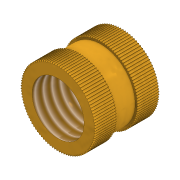
# Autodesk Inventor part: M5 7mm OD 8mm Deep Threaded Insert
Saved by Autodesk Inventor 2020 (Build 240168000, 168)
## iProperties
Created: 2021-07-20
Part Number: M5 7mm OD 8mm Deep Threaded Insert
Material: Generic
Document SubType Name: Modeling
Designer: Coy
Density: 1 g/cm^3
Appearance: Weld - Brass
Author: Coy
Autodesk Inventor part; units mm, degrees
ref_plane "YZ Plane" through (0, 0, 0) normal (1, 0, 0) x (0, 1, 0)
ref_plane "XZ Plane" through (0, 0, 0) normal (0, 1, 0) x (-1, 0, 0)
ref_plane "XY Plane" through (0, 0, 0) normal (0, 0, 1) x (1, 0, 0)
sketch "Sketch1" plane through (0, 0, 0) normal (0, 0, 1) x (1, 0, 0)
  circle A0 centre (0, 0) radius 2.45
  circle A1 centre (0, 0) radius 3.5
  arc A2 (-0.1, 3.4986) -> (0.1, 3.4986) centre (0, 3.5) ccw
  arc A3 (-0.3195, 3.4854) -> (-0.1199, 3.4979) centre (-0.2198, 3.4931) ccw
  arc A4 (-0.5377, 3.4585) -> (-0.3393, 3.4835) centre (-0.4387, 3.4724) ccw
  arc A5 (-0.7538, 3.4179) -> (-0.5573, 3.4553) centre (-0.6558, 3.438) ccw
  arc A6 (-0.9669, 3.3638) -> (-0.7732, 3.4135) centre (-0.8704, 3.39) ccw
  arc A7 (-1.1762, 3.2964) -> (-0.986, 3.3582) centre (-1.0816, 3.3287) ccw
  arc A8 (-1.3809, 3.2161) -> (-1.1949, 3.2897) centre (-1.2884, 3.2542) ccw
  arc A9 (-1.5801, 3.123) -> (-1.3991, 3.2082) centre (-1.4902, 3.1669) ccw
  arc A10 (-1.7731, 3.0177) -> (-1.5978, 3.114) centre (-1.6861, 3.0671) ccw
  arc A11 (-1.9591, 2.9004) -> (-1.7902, 3.0075) centre (-1.8754, 2.9551) ccw
  arc A12 (-2.1373, 2.7716) -> (-1.9755, 2.8892) centre (-2.0572, 2.8316) ccw
  arc A13 (-2.3071, 2.632) -> (-2.153, 2.7594) centre (-2.231, 2.6968) ccw
  arc A14 (-2.4678, 2.4819) -> (-2.322, 2.6188) centre (-2.3959, 2.5514) ccw
  arc A15 (-2.6188, 2.322) -> (-2.4819, 2.4678) centre (-2.5514, 2.3959) ccw
  arc A16 (-2.7594, 2.153) -> (-2.632, 2.3071) centre (-2.6968, 2.231) ccw
  arc A17 (-2.8892, 1.9755) -> (-2.7716, 2.1373) centre (-2.8316, 2.0572) ccw
  arc A18 (-3.0075, 1.7902) -> (-2.9004, 1.9591) centre (-2.9551, 1.8754) ccw
  arc A19 (-3.114, 1.5978) -> (-3.0177, 1.7731) centre (-3.0671, 1.6861) ccw
  arc A20 (-3.2082, 1.3991) -> (-3.123, 1.5801) centre (-3.1669, 1.4902) ccw
  arc A21 (-3.2897, 1.1949) -> (-3.2161, 1.3809) centre (-3.2542, 1.2884) ccw
  arc A22 (-3.3582, 0.986) -> (-3.2964, 1.1762) centre (-3.3287, 1.0816) ccw
  arc A23 (-3.4135, 0.7732) -> (-3.3638, 0.9669) centre (-3.39, 0.8704) ccw
  arc A24 (-3.4553, 0.5573) -> (-3.4179, 0.7538) centre (-3.438, 0.6558) ccw
  arc A25 (-3.4835, 0.3393) -> (-3.4585, 0.5377) centre (-3.4724, 0.4387) ccw
  arc A26 (-3.4979, 0.1199) -> (-3.4854, 0.3195) centre (-3.4931, 0.2198) ccw
  arc A27 (-3.4986, -0.1) -> (-3.4986, 0.1) centre (-3.5, 0) ccw
  arc A28 (-3.4854, -0.3195) -> (-3.4979, -0.1199) centre (-3.4931, -0.2198) ccw
  arc A29 (-3.4585, -0.5377) -> (-3.4835, -0.3393) centre (-3.4724, -0.4387) ccw
  arc A30 (-3.4179, -0.7538) -> (-3.4553, -0.5573) centre (-3.438, -0.6558) ccw
  arc A31 (-3.3638, -0.9669) -> (-3.4135, -0.7732) centre (-3.39, -0.8704) ccw
  arc A32 (-3.2964, -1.1762) -> (-3.3582, -0.986) centre (-3.3287, -1.0816) ccw
  arc A33 (-3.2161, -1.3809) -> (-3.2897, -1.1949) centre (-3.2542, -1.2884) ccw
  arc A34 (-3.123, -1.5801) -> (-3.2082, -1.3991) centre (-3.1669, -1.4902) ccw
  arc A35 (-3.0177, -1.7731) -> (-3.114, -1.5978) centre (-3.0671, -1.6861) ccw
  arc A36 (-2.9004, -1.9591) -> (-3.0075, -1.7902) centre (-2.9551, -1.8754) ccw
  arc A37 (-2.7716, -2.1373) -> (-2.8892, -1.9755) centre (-2.8316, -2.0572) ccw
  arc A38 (-2.632, -2.3071) -> (-2.7594, -2.153) centre (-2.6968, -2.231) ccw
  arc A39 (-2.4819, -2.4678) -> (-2.6188, -2.322) centre (-2.5514, -2.3959) ccw
  arc A40 (-2.322, -2.6188) -> (-2.4678, -2.4819) centre (-2.3959, -2.5514) ccw
  arc A41 (-2.153, -2.7594) -> (-2.3071, -2.632) centre (-2.231, -2.6968) ccw
  arc A42 (-1.9755, -2.8892) -> (-2.1373, -2.7716) centre (-2.0572, -2.8316) ccw
  arc A43 (-1.7902, -3.0075) -> (-1.9591, -2.9004) centre (-1.8754, -2.9551) ccw
  arc A44 (-1.5978, -3.114) -> (-1.7731, -3.0177) centre (-1.6861, -3.0671) ccw
  arc A45 (-1.3991, -3.2082) -> (-1.5801, -3.123) centre (-1.4902, -3.1669) ccw
  arc A46 (-1.1949, -3.2897) -> (-1.3809, -3.2161) centre (-1.2884, -3.2542) ccw
  arc A47 (-0.986, -3.3582) -> (-1.1762, -3.2964) centre (-1.0816, -3.3287) ccw
  arc A48 (-0.7732, -3.4135) -> (-0.9669, -3.3638) centre (-0.8704, -3.39) ccw
  arc A49 (-0.5573, -3.4553) -> (-0.7538, -3.4179) centre (-0.6558, -3.438) ccw
  arc A50 (-0.3393, -3.4835) -> (-0.5377, -3.4585) centre (-0.4387, -3.4724) ccw
  arc A51 (-0.1199, -3.4979) -> (-0.3195, -3.4854) centre (-0.2198, -3.4931) ccw
  arc A52 (0.1, -3.4986) -> (-0.1, -3.4986) centre (0, -3.5) ccw
  arc A53 (0.3195, -3.4854) -> (0.1199, -3.4979) centre (0.2198, -3.4931) ccw
  arc A54 (0.5377, -3.4585) -> (0.3393, -3.4835) centre (0.4387, -3.4724) ccw
  arc A55 (0.7538, -3.4179) -> (0.5573, -3.4553) centre (0.6558, -3.438) ccw
  arc A56 (0.9669, -3.3638) -> (0.7732, -3.4135) centre (0.8704, -3.39) ccw
  arc A57 (1.1762, -3.2964) -> (0.986, -3.3582) centre (1.0816, -3.3287) ccw
  arc A58 (1.3809, -3.2161) -> (1.1949, -3.2897) centre (1.2884, -3.2542) ccw
  arc A59 (1.5801, -3.123) -> (1.3991, -3.2082) centre (1.4902, -3.1669) ccw
  arc A60 (1.7731, -3.0177) -> (1.5978, -3.114) centre (1.6861, -3.0671) ccw
  arc A61 (1.9591, -2.9004) -> (1.7902, -3.0075) centre (1.8754, -2.9551) ccw
  arc A62 (2.1373, -2.7716) -> (1.9755, -2.8892) centre (2.0572, -2.8316) ccw
  arc A63 (2.3071, -2.632) -> (2.153, -2.7594) centre (2.231, -2.6968) ccw
  arc A64 (2.4678, -2.4819) -> (2.322, -2.6188) centre (2.3959, -2.5514) ccw
  arc A65 (2.6188, -2.322) -> (2.4819, -2.4678) centre (2.5514, -2.3959) ccw
  arc A66 (2.7594, -2.153) -> (2.632, -2.3071) centre (2.6968, -2.231) ccw
  arc A67 (2.8892, -1.9755) -> (2.7716, -2.1373) centre (2.8316, -2.0572) ccw
  arc A68 (3.0075, -1.7902) -> (2.9004, -1.9591) centre (2.9551, -1.8754) ccw
  arc A69 (3.114, -1.5978) -> (3.0177, -1.7731) centre (3.0671, -1.6861) ccw
  arc A70 (3.2082, -1.3991) -> (3.123, -1.5801) centre (3.1669, -1.4902) ccw
  arc A71 (3.2897, -1.1949) -> (3.2161, -1.3809) centre (3.2542, -1.2884) ccw
  arc A72 (3.3582, -0.986) -> (3.2964, -1.1762) centre (3.3287, -1.0816) ccw
  arc A73 (3.4135, -0.7732) -> (3.3638, -0.9669) centre (3.39, -0.8704) ccw
  arc A74 (3.4553, -0.5573) -> (3.4179, -0.7538) centre (3.438, -0.6558) ccw
  arc A75 (3.4835, -0.3393) -> (3.4585, -0.5377) centre (3.4724, -0.4387) ccw
  arc A76 (3.4979, -0.1199) -> (3.4854, -0.3195) centre (3.4931, -0.2198) ccw
  arc A77 (3.4986, 0.1) -> (3.4986, -0.1) centre (3.5, 0) ccw
  arc A78 (3.4854, 0.3195) -> (3.4979, 0.1199) centre (3.4931, 0.2198) ccw
  arc A79 (3.4585, 0.5377) -> (3.4835, 0.3393) centre (3.4724, 0.4387) ccw
  arc A80 (3.4179, 0.7538) -> (3.4553, 0.5573) centre (3.438, 0.6558) ccw
  arc A81 (3.3638, 0.9669) -> (3.4135, 0.7732) centre (3.39, 0.8704) ccw
  arc A82 (3.2964, 1.1762) -> (3.3582, 0.986) centre (3.3287, 1.0816) ccw
  arc A83 (3.2161, 1.3809) -> (3.2897, 1.1949) centre (3.2542, 1.2884) ccw
  arc A84 (3.123, 1.5801) -> (3.2082, 1.3991) centre (3.1669, 1.4902) ccw
  arc A85 (3.0177, 1.7731) -> (3.114, 1.5978) centre (3.0671, 1.6861) ccw
  arc A86 (2.9004, 1.9591) -> (3.0075, 1.7902) centre (2.9551, 1.8754) ccw
  arc A87 (2.7716, 2.1373) -> (2.8892, 1.9755) centre (2.8316, 2.0572) ccw
  arc A88 (2.632, 2.3071) -> (2.7594, 2.153) centre (2.6968, 2.231) ccw
  arc A89 (2.4819, 2.4678) -> (2.6188, 2.322) centre (2.5514, 2.3959) ccw
  arc A90 (2.322, 2.6188) -> (2.4678, 2.4819) centre (2.3959, 2.5514) ccw
  arc A91 (2.153, 2.7594) -> (2.3071, 2.632) centre (2.231, 2.6968) ccw
  arc A92 (1.9755, 2.8892) -> (2.1373, 2.7716) centre (2.0572, 2.8316) ccw
  arc A93 (1.7902, 3.0075) -> (1.9591, 2.9004) centre (1.8754, 2.9551) ccw
  arc A94 (1.5978, 3.114) -> (1.7731, 3.0177) centre (1.6861, 3.0671) ccw
  arc A95 (1.3991, 3.2082) -> (1.5801, 3.123) centre (1.4902, 3.1669) ccw
  arc A96 (1.1949, 3.2897) -> (1.3809, 3.2161) centre (1.2884, 3.2542) ccw
  arc A97 (0.986, 3.3582) -> (1.1762, 3.2964) centre (1.0816, 3.3287) ccw
  arc A98 (0.7732, 3.4135) -> (0.9669, 3.3638) centre (0.8704, 3.39) ccw
  arc A99 (0.5573, 3.4553) -> (0.7538, 3.4179) centre (0.6558, 3.438) ccw
  arc A100 (0.3393, 3.4835) -> (0.5377, 3.4585) centre (0.4387, 3.4724) ccw
  arc A101 (0.1199, 3.4979) -> (0.3195, 3.4854) centre (0.2198, 3.4931) ccw
  point P0 (0.3195, 3.4854)
  point P1 (0.1199, 3.4979)
  point P2 (-0.1199, 3.4979)
  point P3 (-0.3195, 3.4854)
  point P4 (-0.3393, 3.4835)
  point P5 (-0.5377, 3.4585)
  point P6 (-0.5573, 3.4553)
  point P7 (-0.9669, 3.3638)
  point P8 (-1.1949, 3.2897)
  point P9 (-1.3991, 3.2082)
  point P10 (-1.5978, 3.114)
  point P11 (-1.9591, 2.9004)
  point P12 (-1.9755, 2.8892)
  point P13 (-2.1373, 2.7716)
  point P14 (-2.153, 2.7594)
  point P15 (-2.4819, 2.4678)
  point P16 (-2.632, 2.3071)
  point P17 (-2.7716, 2.1373)
  point P18 (-2.8892, 1.9755)
  point P19 (-3.0177, 1.7731)
  point P20 (-3.123, 1.5801)
  point P21 (-3.2082, 1.3991)
  point P22 (-3.2964, 1.1762)
  point P23 (-3.3638, 0.9669)
  point P24 (-3.4135, 0.7732)
  point P25 (-3.4179, 0.7538)
  point P26 (-3.4585, 0.5377)
  point P27 (-3.4835, 0.3393)
  point P28 (-3.4854, 0.3195)
  point P29 (-3.4979, 0.1199)
  point P30 (-3.4986, 0.1)
  point P31 (-3.4979, -0.1199)
  point P32 (-3.4835, -0.3393)
  point P33 (-3.4553, -0.5573)
  point P34 (-3.4135, -0.7732)
  point P35 (-3.3638, -0.9669)
  point P36 (-3.2897, -1.1949)
  point P37 (-3.2082, -1.3991)
  point P38 (-2.9004, -1.9591)
  point P39 (-2.8892, -1.9755)
  point P40 (-2.7716, -2.1373)
  point P41 (-2.7594, -2.153)
  point P42 (-2.632, -2.3071)
  point P43 (-2.4678, -2.4819)
  point P44 (-2.153, -2.7594)
  point P45 (-2.1373, -2.7716)
  point P46 (-1.7731, -3.0177)
  point P47 (-1.5801, -3.123)
  point P48 (-1.3991, -3.2082)
  point P49 (-1.3809, -3.2161)
  point P50 (-1.1762, -3.2964)
  point P51 (-0.9669, -3.3638)
  point P52 (-0.7732, -3.4135)
  point P53 (-0.7538, -3.4179)
  point P54 (-0.5377, -3.4585)
  point P55 (-0.3195, -3.4854)
  point P56 (-0.1199, -3.4979)
  point P57 (-0.1, -3.4986)
  point P58 (0.1199, -3.4979)
  point P59 (0.3393, -3.4835)
  point P60 (0.5573, -3.4553)
  point P61 (0.7538, -3.4179)
  point P62 (0.7732, -3.4135)
  point P63 (0.9669, -3.3638)
  point P64 (1.3809, -3.2161)
  point P65 (1.3991, -3.2082)
  point P66 (1.5978, -3.114)
  point P67 (1.9591, -2.9004)
  point P68 (1.9755, -2.8892)
  point P69 (2.153, -2.7594)
  point P70 (2.4819, -2.4678)
  point P71 (2.7594, -2.153)
  point P72 (2.7716, -2.1373)
  point P73 (2.9004, -1.9591)
  point P74 (3.0075, -1.7902)
  point P75 (3.0177, -1.7731)
  point P76 (3.114, -1.5978)
  point P77 (3.123, -1.5801)
  point P78 (3.2897, -1.1949)
  point P79 (3.3638, -0.9669)
  point P80 (3.4135, -0.7732)
  point P81 (3.4179, -0.7538)
  point P82 (3.4585, -0.5377)
  point P83 (3.4854, -0.3195)
  point P84 (3.4979, -0.1199)
  point P85 (3.4986, -0.1)
  point P86 (3.4979, 0.1199)
  point P87 (3.4835, 0.3393)
  point P88 (3.4585, 0.5377)
  point P89 (3.4553, 0.5573)
  point P90 (3.4135, 0.7732)
  point P91 (3.3638, 0.9669)
  point P92 (3.2161, 1.3809)
  point P93 (3.2082, 1.3991)
  point P94 (3.114, 1.5978)
  point P95 (3.0177, 1.7731)
  point P96 (2.9004, 1.9591)
  point P97 (2.8892, 1.9755)
  point P98 (2.7716, 2.1373)
  point P99 (2.7594, 2.153)
  point P100 (2.4819, 2.4678)
  point P101 (1.9755, 2.8892)
  point P102 (1.9591, 2.9004)
  point P103 (1.7902, 3.0075)
  point P104 (1.7731, 3.0177)
  point P105 (1.5978, 3.114)
  point P106 (1.5801, 3.123)
  point P107 (1.1762, 3.2964)
  point P108 (0.9669, 3.3638)
  point P109 (0.7538, 3.4179)
  point P110 (0.5573, 3.4553)
  point P111 (0.5377, 3.4585)
  point P112 (0.3393, 3.4835)
  point P113 (0.3195, 3.4854)
  point P114 (0.1199, 3.4979)
  point P115 (-0.1199, 3.4979)
  point P116 (-0.3195, 3.4854)
  point P117 (-0.3393, 3.4835)
  point P118 (-0.5377, 3.4585)
  point P119 (-0.5573, 3.4553)
  point P120 (-0.9669, 3.3638)
  point P121 (-1.1949, 3.2897)
  point P122 (-1.3991, 3.2082)
  point P123 (-1.5978, 3.114)
  point P124 (-1.9591, 2.9004)
  point P125 (-1.9755, 2.8892)
  point P126 (-2.1373, 2.7716)
  point P127 (-2.153, 2.7594)
  point P128 (-2.4819, 2.4678)
  point P129 (-2.632, 2.3071)
  point P130 (-2.7716, 2.1373)
  point P131 (-2.8892, 1.9755)
  point P132 (-3.0177, 1.7731)
  point P133 (-3.123, 1.5801)
  point P134 (-3.2082, 1.3991)
  point P135 (-3.2964, 1.1762)
  point P136 (-3.3638, 0.9669)
  point P137 (-3.4135, 0.7732)
  point P138 (-3.4179, 0.7538)
  point P139 (-3.4585, 0.5377)
  point P140 (-3.4835, 0.3393)
  point P141 (-3.4854, 0.3195)
  point P142 (-3.4979, 0.1199)
  point P143 (-3.4986, 0.1)
  point P144 (-3.4979, -0.1199)
  point P145 (-3.4835, -0.3393)
  point P146 (-3.4553, -0.5573)
  point P147 (-3.4135, -0.7732)
  point P148 (-3.3638, -0.9669)
  point P149 (-3.2897, -1.1949)
  point P150 (-3.2082, -1.3991)
  point P151 (-2.9004, -1.9591)
  point P152 (-2.8892, -1.9755)
  point P153 (-2.7716, -2.1373)
  point P154 (-2.7594, -2.153)
  point P155 (-2.632, -2.3071)
  point P156 (-2.4678, -2.4819)
  point P157 (-2.153, -2.7594)
  point P158 (-2.1373, -2.7716)
  point P159 (-1.7731, -3.0177)
  point P160 (-1.5801, -3.123)
  point P161 (-1.3991, -3.2082)
  point P162 (-1.3809, -3.2161)
  point P163 (-1.1762, -3.2964)
  point P164 (-0.9669, -3.3638)
  point P165 (-0.7732, -3.4135)
  point P166 (-0.7538, -3.4179)
  point P167 (-0.5377, -3.4585)
  point P168 (-0.3195, -3.4854)
  point P169 (-0.1199, -3.4979)
  point P170 (-0.1, -3.4986)
  point P171 (0.1199, -3.4979)
  point P172 (0.3393, -3.4835)
  point P173 (0.5573, -3.4553)
  point P174 (0.7538, -3.4179)
  point P175 (0.7732, -3.4135)
  point P176 (0.9669, -3.3638)
  point P177 (1.3809, -3.2161)
  point P178 (1.3991, -3.2082)
  point P179 (1.5978, -3.114)
  point P180 (1.9591, -2.9004)
  point P181 (1.9755, -2.8892)
  point P182 (2.153, -2.7594)
  point P183 (2.4819, -2.4678)
  point P184 (2.7594, -2.153)
  point P185 (2.7716, -2.1373)
  point P186 (2.9004, -1.9591)
  point P187 (3.0075, -1.7902)
  point P188 (3.0177, -1.7731)
  point P189 (3.114, -1.5978)
  point P190 (3.123, -1.5801)
  point P191 (3.2897, -1.1949)
  point P192 (3.3638, -0.9669)
  point P193 (3.4135, -0.7732)
  point P194 (3.4179, -0.7538)
  point P195 (3.4585, -0.5377)
  point P196 (3.4854, -0.3195)
  point P197 (3.4979, -0.1199)
  point P198 (3.4986, -0.1)
  point P199 (3.4979, 0.1199)
  dimension "d3" = 7
  dimension "d2" = 4.9
  dimension "d4" = 0.2
  dimension "d5" = 360
  constraints: 200 point on circle, 101 centre point, 2 coincident, 405 other
  measures "d2" diameter of A0
  measures "d4" diameter of A2
extrude "Extrusion1" add sketch "Sketch1" against normal blind 2 contours A77 A1 A76 A75 A74 A73 A72 A71 A70 A69 A68 A67 A66 A65 A64 A63 A62 A61 A60 A59 A58 A57 A56 A55 A54 A53 A52 A51 A50 A49 A48 A47 A46 A45 A44 A43 A42 A41 A40 A39 A38 A37 A36 A35 A34 A33 A32 A31 A30 A29 A28 A27 A26 A25 A24 A23 A22 A21 A20 A19 A18 A17 A16 A15 A14 A13 A12 A11 A10 A9 A8 A7 A6 A5 A4 A3 A2 A101 A100 A99 A98 A97 A96 A95 A94 A93 A92 A91 A90 A89 A88 A87 A86 A85 A84 A83 A82 A81 A80 A79 A78
sketch "Sketch2" plane through (0, 0, -2) normal (0, 0, -1) x (-1, 0, 0)
  circle A0 centre (0, 0) radius 2.45 projected
  circle A1 centre (0, 0) radius 3.25
  dimension "d8" = 6.5
  constraints: 1 centre point, 1 coincident
  measures "d8" diameter of A1
extrude "Extrusion2" add sketch "Sketch2" along normal blind 2
sketch "Sketch3" plane through (0, 0, -4) normal (0, 0, -1) x (-1, 0, 0)
  circle A0 centre (0, 0) radius 3.25 projected
  arc A1 (1.1949, 3.2897) -> (1.1762, 3.2964) centre (0, 0) ccw projected
  arc A2 (0.986, 3.3582) -> (1.1762, 3.2964) centre (1.0816, 3.3287) ccw projected
  arc A3 (0.986, 3.3582) -> (0.9669, 3.3638) centre (0, 0) ccw projected
  arc A4 (0.7732, 3.4135) -> (0.9669, 3.3638) centre (0.8704, 3.39) ccw projected
  arc A5 (0.7732, 3.4135) -> (0.7538, 3.4179) centre (0, 0) ccw projected
  arc A6 (0.5573, 3.4553) -> (0.7538, 3.4179) centre (0.6558, 3.438) ccw projected
  arc A7 (0.5573, 3.4553) -> (0.5377, 3.4585) centre (0, 0) ccw projected
  arc A8 (0.3393, 3.4835) -> (0.5377, 3.4585) centre (0.4387, 3.4724) ccw projected
  arc A9 (0.3393, 3.4835) -> (0.3195, 3.4854) centre (0, 0) ccw projected
  arc A10 (0.1199, 3.4979) -> (0.3195, 3.4854) centre (0.2198, 3.4931) ccw projected
  arc A11 (0.1199, 3.4979) -> (0.1, 3.4986) centre (0, 0) ccw projected
  arc A12 (-0.1, 3.4986) -> (0.1, 3.4986) centre (0, 3.5) ccw projected
  arc A13 (-0.1, 3.4986) -> (-0.1199, 3.4979) centre (0, 0) ccw projected
  arc A14 (-0.3195, 3.4854) -> (-0.1199, 3.4979) centre (-0.2198, 3.4931) ccw projected
  arc A15 (-0.3195, 3.4854) -> (-0.3393, 3.4835) centre (0, 0) ccw projected
  arc A16 (-0.5377, 3.4585) -> (-0.3393, 3.4835) centre (-0.4387, 3.4724) ccw projected
  arc A17 (-0.5377, 3.4585) -> (-0.5573, 3.4553) centre (0, 0) ccw projected
  arc A18 (-0.7538, 3.4179) -> (-0.5573, 3.4553) centre (-0.6558, 3.438) ccw projected
  arc A19 (-0.7538, 3.4179) -> (-0.7732, 3.4135) centre (0, 0) ccw projected
  arc A20 (-0.9669, 3.3638) -> (-0.7732, 3.4135) centre (-0.8704, 3.39) ccw projected
  arc A21 (-0.9669, 3.3638) -> (-0.986, 3.3582) centre (0, 0) ccw projected
  arc A22 (-1.1762, 3.2964) -> (-0.986, 3.3582) centre (-1.0816, 3.3287) ccw projected
  arc A23 (-1.1762, 3.2964) -> (-1.1949, 3.2897) centre (0, 0) ccw projected
  arc A24 (-1.3809, 3.2161) -> (-1.1949, 3.2897) centre (-1.2884, 3.2542) ccw projected
  arc A25 (-1.3809, 3.2161) -> (-1.3991, 3.2082) centre (0, 0) ccw projected
  arc A26 (-1.5801, 3.123) -> (-1.3991, 3.2082) centre (-1.4902, 3.1669) ccw projected
  arc A27 (-1.5801, 3.123) -> (-1.5978, 3.114) centre (0, 0) ccw projected
  arc A28 (-1.7731, 3.0177) -> (-1.5978, 3.114) centre (-1.6861, 3.0671) ccw projected
  arc A29 (-1.7731, 3.0177) -> (-1.7902, 3.0075) centre (0, 0) ccw projected
  arc A30 (-1.9591, 2.9004) -> (-1.7902, 3.0075) centre (-1.8754, 2.9551) ccw projected
  arc A31 (-1.9591, 2.9004) -> (-1.9755, 2.8892) centre (0, 0) ccw projected
  arc A32 (-2.1373, 2.7716) -> (-1.9755, 2.8892) centre (-2.0572, 2.8316) ccw projected
  arc A33 (-2.1373, 2.7716) -> (-2.153, 2.7594) centre (0, 0) ccw projected
  arc A34 (-2.3071, 2.632) -> (-2.153, 2.7594) centre (-2.231, 2.6968) ccw projected
  arc A35 (-2.3071, 2.632) -> (-2.322, 2.6188) centre (0, 0) ccw projected
  arc A36 (-2.4678, 2.4819) -> (-2.322, 2.6188) centre (-2.3959, 2.5514) ccw projected
  arc A37 (-2.4678, 2.4819) -> (-2.4819, 2.4678) centre (0, 0) ccw projected
  arc A38 (-2.6188, 2.322) -> (-2.4819, 2.4678) centre (-2.5514, 2.3959) ccw projected
  arc A39 (-2.6188, 2.322) -> (-2.632, 2.3071) centre (0, 0) ccw projected
  arc A40 (-2.7594, 2.153) -> (-2.632, 2.3071) centre (-2.6968, 2.231) ccw projected
  arc A41 (-2.7594, 2.153) -> (-2.7716, 2.1373) centre (0, 0) ccw projected
  arc A42 (-2.8892, 1.9755) -> (-2.7716, 2.1373) centre (-2.8316, 2.0572) ccw projected
  arc A43 (-2.8892, 1.9755) -> (-2.9004, 1.9591) centre (0, 0) ccw projected
  arc A44 (-3.0075, 1.7902) -> (-2.9004, 1.9591) centre (-2.9551, 1.8754) ccw projected
  arc A45 (-3.0075, 1.7902) -> (-3.0177, 1.7731) centre (0, 0) ccw projected
  arc A46 (-3.114, 1.5978) -> (-3.0177, 1.7731) centre (-3.0671, 1.6861) ccw projected
  arc A47 (-3.114, 1.5978) -> (-3.123, 1.5801) centre (0, 0) ccw projected
  arc A48 (-3.2082, 1.3991) -> (-3.123, 1.5801) centre (-3.1669, 1.4902) ccw projected
  arc A49 (-3.2082, 1.3991) -> (-3.2161, 1.3809) centre (0, 0) ccw projected
  arc A50 (-3.2897, 1.1949) -> (-3.2161, 1.3809) centre (-3.2542, 1.2884) ccw projected
  arc A51 (-3.2897, 1.1949) -> (-3.2964, 1.1762) centre (0, 0) ccw projected
  arc A52 (-3.3582, 0.986) -> (-3.2964, 1.1762) centre (-3.3287, 1.0816) ccw projected
  arc A53 (-3.3582, 0.986) -> (-3.3638, 0.9669) centre (0, 0) ccw projected
  arc A54 (-3.4135, 0.7732) -> (-3.3638, 0.9669) centre (-3.39, 0.8704) ccw projected
  arc A55 (-3.4135, 0.7732) -> (-3.4179, 0.7538) centre (0, 0) ccw projected
  arc A56 (-3.4553, 0.5573) -> (-3.4179, 0.7538) centre (-3.438, 0.6558) ccw projected
  arc A57 (-3.4553, 0.5573) -> (-3.4585, 0.5377) centre (0, 0) ccw projected
  arc A58 (-3.4835, 0.3393) -> (-3.4585, 0.5377) centre (-3.4724, 0.4387) ccw projected
  arc A59 (-3.4835, 0.3393) -> (-3.4854, 0.3195) centre (0, 0) ccw projected
  arc A60 (-3.4979, 0.1199) -> (-3.4854, 0.3195) centre (-3.4931, 0.2198) ccw projected
  arc A61 (-3.4979, 0.1199) -> (-3.4986, 0.1) centre (0, 0) ccw projected
  arc A62 (-3.4986, -0.1) -> (-3.4986, 0.1) centre (-3.5, 0) ccw projected
  arc A63 (-3.4986, -0.1) -> (-3.4979, -0.1199) centre (0, 0) ccw projected
  arc A64 (-3.4854, -0.3195) -> (-3.4979, -0.1199) centre (-3.4931, -0.2198) ccw projected
  arc A65 (-3.4854, -0.3195) -> (-3.4835, -0.3393) centre (0, 0) ccw projected
  arc A66 (-3.4585, -0.5377) -> (-3.4835, -0.3393) centre (-3.4724, -0.4387) ccw projected
  arc A67 (-3.4585, -0.5377) -> (-3.4553, -0.5573) centre (0, 0) ccw projected
  arc A68 (-3.4179, -0.7538) -> (-3.4553, -0.5573) centre (-3.438, -0.6558) ccw projected
  arc A69 (-3.4179, -0.7538) -> (-3.4135, -0.7732) centre (0, 0) ccw projected
  arc A70 (-3.3638, -0.9669) -> (-3.4135, -0.7732) centre (-3.39, -0.8704) ccw projected
  arc A71 (-3.3638, -0.9669) -> (-3.3582, -0.986) centre (0, 0) ccw projected
  arc A72 (-3.2964, -1.1762) -> (-3.3582, -0.986) centre (-3.3287, -1.0816) ccw projected
  arc A73 (-3.2964, -1.1762) -> (-3.2897, -1.1949) centre (0, 0) ccw projected
  arc A74 (-3.2161, -1.3809) -> (-3.2897, -1.1949) centre (-3.2542, -1.2884) ccw projected
  arc A75 (-3.2161, -1.3809) -> (-3.2082, -1.3991) centre (0, 0) ccw projected
  arc A76 (-3.123, -1.5801) -> (-3.2082, -1.3991) centre (-3.1669, -1.4902) ccw projected
  arc A77 (-3.123, -1.5801) -> (-3.114, -1.5978) centre (0, 0) ccw projected
  arc A78 (-3.0177, -1.7731) -> (-3.114, -1.5978) centre (-3.0671, -1.6861) ccw projected
  arc A79 (-3.0177, -1.7731) -> (-3.0075, -1.7902) centre (0, 0) ccw projected
  arc A80 (-2.9004, -1.9591) -> (-3.0075, -1.7902) centre (-2.9551, -1.8754) ccw projected
  arc A81 (-2.9004, -1.9591) -> (-2.8892, -1.9755) centre (0, 0) ccw projected
  arc A82 (-2.7716, -2.1373) -> (-2.8892, -1.9755) centre (-2.8316, -2.0572) ccw projected
  arc A83 (-2.7716, -2.1373) -> (-2.7594, -2.153) centre (0, 0) ccw projected
  arc A84 (-2.632, -2.3071) -> (-2.7594, -2.153) centre (-2.6968, -2.231) ccw projected
  arc A85 (-2.632, -2.3071) -> (-2.6188, -2.322) centre (0, 0) ccw projected
  arc A86 (-2.4819, -2.4678) -> (-2.6188, -2.322) centre (-2.5514, -2.3959) ccw projected
  arc A87 (-2.4819, -2.4678) -> (-2.4678, -2.4819) centre (0, 0) ccw projected
  arc A88 (-2.322, -2.6188) -> (-2.4678, -2.4819) centre (-2.3959, -2.5514) ccw projected
  arc A89 (-2.322, -2.6188) -> (-2.3071, -2.632) centre (0, 0) ccw projected
  arc A90 (-2.153, -2.7594) -> (-2.3071, -2.632) centre (-2.231, -2.6968) ccw projected
  arc A91 (-2.153, -2.7594) -> (-2.1373, -2.7716) centre (0, 0) ccw projected
  arc A92 (-1.9755, -2.8892) -> (-2.1373, -2.7716) centre (-2.0572, -2.8316) ccw projected
  arc A93 (-1.9755, -2.8892) -> (-1.9591, -2.9004) centre (0, 0) ccw projected
  arc A94 (-1.7902, -3.0075) -> (-1.9591, -2.9004) centre (-1.8754, -2.9551) ccw projected
  arc A95 (-1.7902, -3.0075) -> (-1.7731, -3.0177) centre (0, 0) ccw projected
  arc A96 (-1.5978, -3.114) -> (-1.7731, -3.0177) centre (-1.6861, -3.0671) ccw projected
  arc A97 (-1.5978, -3.114) -> (-1.5801, -3.123) centre (0, 0) ccw projected
  arc A98 (-1.3991, -3.2082) -> (-1.5801, -3.123) centre (-1.4902, -3.1669) ccw projected
  arc A99 (-1.3991, -3.2082) -> (-1.3809, -3.2161) centre (0, 0) ccw projected
  arc A100 (-1.1949, -3.2897) -> (-1.3809, -3.2161) centre (-1.2884, -3.2542) ccw projected
  arc A101 (-1.1949, -3.2897) -> (-1.1762, -3.2964) centre (0, 0) ccw projected
  arc A102 (-0.986, -3.3582) -> (-1.1762, -3.2964) centre (-1.0816, -3.3287) ccw projected
  arc A103 (-0.986, -3.3582) -> (-0.9669, -3.3638) centre (0, 0) ccw projected
  arc A104 (-0.7732, -3.4135) -> (-0.9669, -3.3638) centre (-0.8704, -3.39) ccw projected
  arc A105 (-0.7732, -3.4135) -> (-0.7538, -3.4179) centre (0, 0) ccw projected
  arc A106 (-0.5573, -3.4553) -> (-0.7538, -3.4179) centre (-0.6558, -3.438) ccw projected
  arc A107 (-0.5573, -3.4553) -> (-0.5377, -3.4585) centre (0, 0) ccw projected
  arc A108 (-0.3393, -3.4835) -> (-0.5377, -3.4585) centre (-0.4387, -3.4724) ccw projected
  arc A109 (-0.3393, -3.4835) -> (-0.3195, -3.4854) centre (0, 0) ccw projected
  arc A110 (-0.1199, -3.4979) -> (-0.3195, -3.4854) centre (-0.2198, -3.4931) ccw projected
  arc A111 (-0.1199, -3.4979) -> (-0.1, -3.4986) centre (0, 0) ccw projected
  arc A112 (0.1, -3.4986) -> (-0.1, -3.4986) centre (0, -3.5) ccw projected
  arc A113 (0.1, -3.4986) -> (0.1199, -3.4979) centre (0, 0) ccw projected
  arc A114 (0.3195, -3.4854) -> (0.1199, -3.4979) centre (0.2198, -3.4931) ccw projected
  arc A115 (0.3195, -3.4854) -> (0.3393, -3.4835) centre (0, 0) ccw projected
  arc A116 (0.5377, -3.4585) -> (0.3393, -3.4835) centre (0.4387, -3.4724) ccw projected
  arc A117 (0.5377, -3.4585) -> (0.5573, -3.4553) centre (0, 0) ccw projected
  arc A118 (0.7538, -3.4179) -> (0.5573, -3.4553) centre (0.6558, -3.438) ccw projected
  arc A119 (0.7538, -3.4179) -> (0.7732, -3.4135) centre (0, 0) ccw projected
  arc A120 (0.9669, -3.3638) -> (0.7732, -3.4135) centre (0.8704, -3.39) ccw projected
  arc A121 (0.9669, -3.3638) -> (0.986, -3.3582) centre (0, 0) ccw projected
  arc A122 (1.1762, -3.2964) -> (0.986, -3.3582) centre (1.0816, -3.3287) ccw projected
  arc A123 (1.1762, -3.2964) -> (1.1949, -3.2897) centre (0, 0) ccw projected
  arc A124 (1.3809, -3.2161) -> (1.1949, -3.2897) centre (1.2884, -3.2542) ccw projected
  arc A125 (1.3809, -3.2161) -> (1.3991, -3.2082) centre (0, 0) ccw projected
  arc A126 (1.5801, -3.123) -> (1.3991, -3.2082) centre (1.4902, -3.1669) ccw projected
  arc A127 (1.5801, -3.123) -> (1.5978, -3.114) centre (0, 0) ccw projected
  arc A128 (1.7731, -3.0177) -> (1.5978, -3.114) centre (1.6861, -3.0671) ccw projected
  arc A129 (1.7731, -3.0177) -> (1.7902, -3.0075) centre (0, 0) ccw projected
  arc A130 (1.9591, -2.9004) -> (1.7902, -3.0075) centre (1.8754, -2.9551) ccw projected
  arc A131 (1.9591, -2.9004) -> (1.9755, -2.8892) centre (0, 0) ccw projected
  arc A132 (2.1373, -2.7716) -> (1.9755, -2.8892) centre (2.0572, -2.8316) ccw projected
  arc A133 (2.1373, -2.7716) -> (2.153, -2.7594) centre (0, 0) ccw projected
  arc A134 (2.3071, -2.632) -> (2.153, -2.7594) centre (2.231, -2.6968) ccw projected
  arc A135 (2.3071, -2.632) -> (2.322, -2.6188) centre (0, 0) ccw projected
  arc A136 (2.4678, -2.4819) -> (2.322, -2.6188) centre (2.3959, -2.5514) ccw projected
  arc A137 (2.4678, -2.4819) -> (2.4819, -2.4678) centre (0, 0) ccw projected
  arc A138 (2.6188, -2.322) -> (2.4819, -2.4678) centre (2.5514, -2.3959) ccw projected
  arc A139 (2.6188, -2.322) -> (2.632, -2.3071) centre (0, 0) ccw projected
  arc A140 (2.7594, -2.153) -> (2.632, -2.3071) centre (2.6968, -2.231) ccw projected
  arc A141 (2.7594, -2.153) -> (2.7716, -2.1373) centre (0, 0) ccw projected
  arc A142 (2.8892, -1.9755) -> (2.7716, -2.1373) centre (2.8316, -2.0572) ccw projected
  arc A143 (2.8892, -1.9755) -> (2.9004, -1.9591) centre (0, 0) ccw projected
  arc A144 (3.0075, -1.7902) -> (2.9004, -1.9591) centre (2.9551, -1.8754) ccw projected
  arc A145 (3.0075, -1.7902) -> (3.0177, -1.7731) centre (0, 0) ccw projected
  arc A146 (3.114, -1.5978) -> (3.0177, -1.7731) centre (3.0671, -1.6861) ccw projected
  arc A147 (3.114, -1.5978) -> (3.123, -1.5801) centre (0, 0) ccw projected
  arc A148 (3.2082, -1.3991) -> (3.123, -1.5801) centre (3.1669, -1.4902) ccw projected
  arc A149 (3.2082, -1.3991) -> (3.2161, -1.3809) centre (0, 0) ccw projected
  arc A150 (3.2897, -1.1949) -> (3.2161, -1.3809) centre (3.2542, -1.2884) ccw projected
  arc A151 (3.2897, -1.1949) -> (3.2964, -1.1762) centre (0, 0) ccw projected
  arc A152 (3.3582, -0.986) -> (3.2964, -1.1762) centre (3.3287, -1.0816) ccw projected
  arc A153 (3.3582, -0.986) -> (3.3638, -0.9669) centre (0, 0) ccw projected
  arc A154 (3.4135, -0.7732) -> (3.3638, -0.9669) centre (3.39, -0.8704) ccw projected
  arc A155 (3.4135, -0.7732) -> (3.4179, -0.7538) centre (0, 0) ccw projected
  arc A156 (3.4553, -0.5573) -> (3.4179, -0.7538) centre (3.438, -0.6558) ccw projected
  arc A157 (3.4553, -0.5573) -> (3.4585, -0.5377) centre (0, 0) ccw projected
  arc A158 (3.4835, -0.3393) -> (3.4585, -0.5377) centre (3.4724, -0.4387) ccw projected
  arc A159 (3.4835, -0.3393) -> (3.4854, -0.3195) centre (0, 0) ccw projected
  arc A160 (3.4979, -0.1199) -> (3.4854, -0.3195) centre (3.4931, -0.2198) ccw projected
  arc A161 (3.4979, -0.1199) -> (3.4986, -0.1) centre (0, 0) ccw projected
  arc A162 (3.4986, 0.1) -> (3.4986, -0.1) centre (3.5, 0) ccw projected
  arc A163 (3.4986, 0.1) -> (3.4979, 0.1199) centre (0, 0) ccw projected
  arc A164 (3.4854, 0.3195) -> (3.4979, 0.1199) centre (3.4931, 0.2198) ccw projected
  arc A165 (3.4854, 0.3195) -> (3.4835, 0.3393) centre (0, 0) ccw projected
  arc A166 (3.4585, 0.5377) -> (3.4835, 0.3393) centre (3.4724, 0.4387) ccw projected
  arc A167 (3.4585, 0.5377) -> (3.4553, 0.5573) centre (0, 0) ccw projected
  arc A168 (3.4179, 0.7538) -> (3.4553, 0.5573) centre (3.438, 0.6558) ccw projected
  arc A169 (3.4179, 0.7538) -> (3.4135, 0.7732) centre (0, 0) ccw projected
  arc A170 (3.3638, 0.9669) -> (3.4135, 0.7732) centre (3.39, 0.8704) ccw projected
  arc A171 (3.3638, 0.9669) -> (3.3582, 0.986) centre (0, 0) ccw projected
  arc A172 (3.2964, 1.1762) -> (3.3582, 0.986) centre (3.3287, 1.0816) ccw projected
  arc A173 (3.2964, 1.1762) -> (3.2897, 1.1949) centre (0, 0) ccw projected
  arc A174 (3.2161, 1.3809) -> (3.2897, 1.1949) centre (3.2542, 1.2884) ccw projected
  arc A175 (3.2161, 1.3809) -> (3.2082, 1.3991) centre (0, 0) ccw projected
  arc A176 (3.123, 1.5801) -> (3.2082, 1.3991) centre (3.1669, 1.4902) ccw projected
  arc A177 (3.123, 1.5801) -> (3.114, 1.5978) centre (0, 0) ccw projected
  arc A178 (3.0177, 1.7731) -> (3.114, 1.5978) centre (3.0671, 1.6861) ccw projected
  arc A179 (3.0177, 1.7731) -> (3.0075, 1.7902) centre (0, 0) ccw projected
  arc A180 (2.9004, 1.9591) -> (3.0075, 1.7902) centre (2.9551, 1.8754) ccw projected
  arc A181 (2.9004, 1.9591) -> (2.8892, 1.9755) centre (0, 0) ccw projected
  arc A182 (2.7716, 2.1373) -> (2.8892, 1.9755) centre (2.8316, 2.0572) ccw projected
  arc A183 (2.7716, 2.1373) -> (2.7594, 2.153) centre (0, 0) ccw projected
  arc A184 (2.632, 2.3071) -> (2.7594, 2.153) centre (2.6968, 2.231) ccw projected
  arc A185 (2.632, 2.3071) -> (2.6188, 2.322) centre (0, 0) ccw projected
  arc A186 (2.4819, 2.4678) -> (2.6188, 2.322) centre (2.5514, 2.3959) ccw projected
  arc A187 (2.4819, 2.4678) -> (2.4678, 2.4819) centre (0, 0) ccw projected
  arc A188 (2.322, 2.6188) -> (2.4678, 2.4819) centre (2.3959, 2.5514) ccw projected
  arc A189 (2.322, 2.6188) -> (2.3071, 2.632) centre (0, 0) ccw projected
  arc A190 (2.153, 2.7594) -> (2.3071, 2.632) centre (2.231, 2.6968) ccw projected
  arc A191 (2.153, 2.7594) -> (2.1373, 2.7716) centre (0, 0) ccw projected
  arc A192 (1.9755, 2.8892) -> (2.1373, 2.7716) centre (2.0572, 2.8316) ccw projected
  arc A193 (1.9755, 2.8892) -> (1.9591, 2.9004) centre (0, 0) ccw projected
  arc A194 (1.7902, 3.0075) -> (1.9591, 2.9004) centre (1.8754, 2.9551) ccw projected
  arc A195 (1.7902, 3.0075) -> (1.7731, 3.0177) centre (0, 0) ccw projected
  arc A196 (1.5978, 3.114) -> (1.7731, 3.0177) centre (1.6861, 3.0671) ccw projected
  arc A197 (1.5978, 3.114) -> (1.5801, 3.123) centre (0, 0) ccw projected
  arc A198 (1.3991, 3.2082) -> (1.5801, 3.123) centre (1.4902, 3.1669) ccw projected
  arc A199 (1.3991, 3.2082) -> (1.3809, 3.2161) centre (0, 0) ccw projected
  arc A200 (1.1949, 3.2897) -> (1.3809, 3.2161) centre (1.2884, 3.2542) ccw projected
  circle A201 centre (0, 0) radius 3.25 projected
  circle A202 centre (0, 0) radius 2.45 projected
extrude "Extrusion3" add sketch "Sketch3" along normal blind 2 contours A0 | A200 A199 A198 A197 A196 A195 A194 A193 A192 A191 A190 A189 A188 A187 A186 A185 A184 A183 A182 A181 A180 A179 A178 A177 A176 A175 A174 A173 A172 A171 A170 A169 A168 A167 A166 A165 A164 A163 A162 A161 A160 A159 A158 A157 A156 A155 A154 A153 A152 A151 A150 A149 A148 A147 A146 A145 A144 A143 A142 A141 A140 A139 A138 A137 A136 A135 A134 A133 A132 A131 A130 A129 A128 A127 A126 A125 A124 A123 A122 A121 A120 A119 A118 A117 A116 A115 A114 A113 A112 A111 A110 A109 A108 A107 A106 A105 A104 A103 A102 A101 A100 A99 A98 A97 A96 A95 A94 A93 A92 A91 A90 A89 A88 A87 A86 A85 A84 A83 A82 A81 A80 A79 A78 A77 A76 A75 A74 A73 A72 A71 A70 A69 A68 A67 A66 A65 A64 A63 A62 A61 A60 A59 A58 A57 A56 A55 A54 A53 A52 A51 A50 A49 A48 A47 A46 A45 A44 A43 A42 A41 A40 A39 A38 A37 A36 A35 A34 A33 A32 A31 A30 A29 A28 A27 A26 A25 A24 A23 A22 A21 A20 A19 A18 A17 A16 A15 A14 A13 A12 A11 A10 A9 A8 A7 A6 A5 A4 A3 A2 A1
thread "Thread1" size "M5x0.8" class "6H" standard "ANSI Metric M Profile" full length
body "Solid1"
